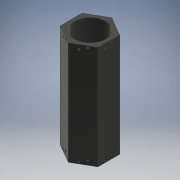
# Autodesk Inventor part: A01
Saved by Autodesk Inventor 2017 SP1 (Build 210196100, 196)
## iProperties
Created: 2019-09-19
Part Number: A01
Material: ABS Plastic
Document SubType Name: Modeling
Designer: Dell
Density: 1.06 g/cm^3
Appearance: Smooth - Black
Mass: 409.304 g
Surface Area: 1165.04 cm^2
Volume: 386.136 cm^3
Author: Dell
Autodesk Inventor part; units mm, degrees
ref_plane "YZ Plane" through (0, 0, 0) normal (1, 0, 0) x (0, 1, 0)
ref_plane "XZ Plane" through (0, 0, 0) normal (0, 1, 0) x (-1, 0, 0)
ref_plane "XY Plane" through (0, 0, 0) normal (0, 0, 1) x (1, 0, 0)
sketch "Sketch1" plane through (0, 0, 0) normal (0, 0, 1) x (1, 0, 0)
  line L0 (0, 46.188) -> (40, 23.094)
  line L1 (40, 23.094) -> (40, -23.094)
  line L2 (40, -23.094) -> (0, -46.188)
  line L3 (0, -46.188) -> (-40, -23.094)
  line L4 (-40, -23.094) -> (-40, 23.094)
  line L5 (-40, 23.094) -> (0, 46.188)
  line L6 (0, 38.1051) -> (33, 19.0526)
  line L7 (33, 19.0526) -> (33, -19.0526)
  line L8 (33, -19.0526) -> (0, -38.1051)
  line L9 (0, -38.1051) -> (-33, -19.0526)
  line L10 (-33, -19.0526) -> (-33, 19.0526)
  line L11 (-33, 19.0526) -> (0, 38.1051)
  point P0 (0, 0)
  point P1 (0, 0)
  dimension "d1" = 66
  dimension "d36" = 7
  constraints: 24 end point, 1 coincident, 1 vertical alignment, 18 other
  measures "d1" distance between parallel lines of L7 L10
  measures "d36" distance between parallel lines of L1 L7
extrude "Extrusion1" add sketch "Sketch1" along normal blind 220
sketch "Sketch2" plane through (40, -23.094, 0) normal (1, 0, 0) x (0, 0, -1)
  line L0 (-211, 16.0229) -> (-216, 30.1651) construction
  line L1 (-220, 0) -> (-220, 46.188) projected
  circle A0 centre (-216, 30.1651) radius 2.5
  circle A1 centre (-211, 16.0229) radius 2.5
  line L2 (-4, 16.0229) -> (-9, 30.1651) construction
  circle A2 centre (-9, 30.1651) radius 2.5
  circle A3 centre (-4, 16.0229) radius 2.5
  line L3 (0, 46.188) -> (0, 0) projected
  point P0 (0, 23.094)
  point P1 (-213.5, 23.094)
  point P2 (-220, 23.094)
  point P3 (-6.5, 23.094)
  point P4 (0, 23.094)
  dimension "d4" = 15
  dimension "d6" = 5
  dimension "d7" = 5
  dimension "d28" = 6.5
  dimension "d29" = 5
  dimension "d30" = 15
  dimension "d31" = 5
  dimension "d32" = 5
  dimension "d34" = 5
  dimension "d35" = 6.5
  constraints: 4 centre point, 4 coincident, 4 end point, 4 midpoint, 2 horizontal alignment
  measures "d4" distance of L0.start L0.end
  measures "d6" diameter of A0
  measures "d7" diameter of A1
  measures "d28" distance of point (-220, 23.094) point (-213.5, 23.094)
  measures "d29" horizontal distance of L0.start L0.end
  measures "d30" distance of L2.start L2.end
  measures "d31" diameter of A2
  measures "d32" diameter of A3
  measures "d34" horizontal distance of L2.start L2.end
  measures "d35" distance of point (0, 23.094) point (-6.5, 23.094)
extrude "Extrusion2" cut sketch "Sketch2" against normal blind 30
pattern_circular "Circular Pattern1" count 6 over 360 about axis through (0, 0, -10) along (0, 0, 1) of "Extrusion2"
sketch "Sketch7" plane through (0, 0, 220) normal (0, 0, 1) x (1, 0, 0)
  circle A0 centre (0, 0) radius 33
  line L0 (-33, 19.0526) -> (0, 38.1051) projected
  line L1 (33, 19.0526) -> (33, -19.0526) projected
  line L2 (33, -19.0526) -> (0, -38.1051) projected
  line L3 (0, -38.1051) -> (-33, -19.0526) projected
  line L4 (-33, -19.0526) -> (-33, 19.0526) projected
  line L5 (-33, 19.0526) -> (0, 38.1051) projected
  line L6 (0, 38.1051) -> (33, 19.0526) projected
  line L7 (40, 23.094) -> (0, 46.188) projected
  line L8 (0, 46.188) -> (-40, 23.094) projected
  line L9 (-40, 23.094) -> (-40, -23.094) projected
  line L10 (-40, -23.094) -> (0, -46.188) projected
  line L11 (0, -46.188) -> (40, -23.094) projected
  line L12 (40, -23.094) -> (40, 23.094) projected
  constraints: 1 centre point, 1 coincident, 1 tangent
extrude "Extrusion6" add sketch "Sketch7" against normal up to surface (220 mm away) from surface at 0 contours L1 L2 A0 | A0 L6 L1 | A0 L0 L6 | L2 L3 A0 | A0 L4 L0 | L3 L4 A0
body "Solid1"
